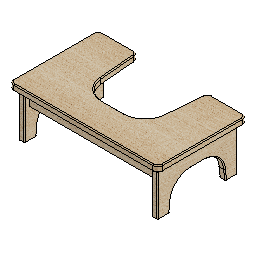
model (Autodesk Fusion 360 design; units mm, degrees)
Autodesk Fusion 360 part; units mm, degrees
sketch "top" plane through (0, 0, 0) normal (0, 0, 1) x (1, 0, 0) in component "stool"
  line L0 (0, 0) -> (500, 0)
  line L1 (150, 100.7611) -> (132.5689, 300)
  line L2 (132.5689, 300) -> (0, 300)
  line L3 (0, 300) -> (0, 0)
  line L4 (150, 100.7611) -> (350, 100.7611)
  line L5 (500, 300) -> (500, 0)
  line L6 (350, 100.7611) -> (367.4311, 300)
  line L7 (367.4311, 300) -> (500, 300)
  arc A0 (285.8568, 100.7611) -> (355.5904, 164.6602) centre (285.8568, 170.7611) ccw
  arc A1 (144.4096, 164.6602) -> (214.1432, 100.7611) centre (214.1432, 170.7611) ccw
  dimension "d5" = 300
  dimension "d6" = 500
  dimension "d7" = 200
  dimension "d8" = 200
  dimension "d21" = 70
  dimension "d36" = 95
  dimension "d37" = 95
  constraint horizontal L0
  constraint horizontal L2
  constraint vertical L3
  constraint coincident L0.start L3.end
  constraint horizontal L4
  constraint vertical L5
  constraint horizontal L7
  constraint equal L2 L7
  constraint equal L3 L5
  constraint tangent L4 A0
  constraint coincident L4 A0.start
  constraint coincident L6 A0.end
  constraint tangent L1 A1
  constraint coincident L1 A1.start
  constraint coincident L4 A1.end
  constraint tangent L6 A0
  constraint tangent L4 A1
  constraint equal A0 A1
  measures "d5" distance of L0.start L2.end
  measures "d6" distance of L0.start L0.end
  measures "d7" distance of L1.start L4.end
  measures "d8" distance of L1.end L1.start
  measures "d21" radius of A0
  measures "d36" angle of L6 L7
  measures "d37" angle of L1 L2
extrude "Extrude1" add sketch "top" along normal blind 21 makes body 1 in component "stool"
sketch "side" plane through (0, 0, 0) normal (1, 0, 0) x (0, 1, 0) in component "stool"
  line L0 (284, 0) -> (284, -150)
  line L1 (284, -150) -> (244, -150)
  line L2 (244, -150) -> (241.0166, -115.8991)
  arc A0 (241.0166, -115.8991) -> (171.2829, -52) centre (171.2829, -122) ccw
  line L3 (171.2829, -52) -> (128.7171, -52)
  arc A1 (128.7171, -52) -> (58.9834, -115.8991) centre (128.7171, -122) ccw
  line L4 (58.9834, -115.8991) -> (56, -150)
  line L5 (56, -150) -> (16, -150)
  line L6 (16, -150) -> (16, 0)
  line L7 (284, 0) -> (16, 0)
  line L8 (150, -52) -> (150, 0) construction
  line L9 (16, 0) -> (0, 0) construction
  point P0 (300, 0)
  dimension "d13" = 16
  dimension "d14" = 16
  dimension "d15" = 40
  dimension "d17" = 150
  dimension "d18" = 70
  dimension "d32" = 52
  dimension "d34" = 95
  dimension "d35" = 95
  constraint tangent L2 A0
  constraint tangent A0 L3
  constraint tangent L3 A1
  constraint tangent A1 L4
  constraint vertical L0
  constraint horizontal L1
  constraint horizontal L3
  constraint horizontal L5
  constraint vertical L6
  constraint equal L1 L5
  constraint equal L0 L6
  constraint equal A0 A1
  constraint perpendicular L6 L7
  constraint midpoint L3 L8.start
  constraint midpoint L7 L8.end
  constraint coincident L9.end origin
  constraint horizontal L9.end L6.end
  measures "d13" distance of P0 L0.start
  measures "d14" distance of L9.end L6.end
  measures "d15" distance of L0.end L1.end
  measures "d17" distance of L0.start L0.end
  measures "d18" radius of A0
  measures "d32" distance of L8.start L8.end
  measures "d34" angle of L1 L2
  measures "d35" angle of L4 L5
extrude "Extrude2" add sketch "side" along normal blind 21 from surface at 16 separate body makes body 2 in component "stool"
ref_plane "WorkPlane1" through (250, 150, 10.5) normal (-1, 0, 0) x (0, -1, 0) in component "stool"
mirror "Mirror1" about plane through (250, 150, 10.5) normal (-1, 0, 0) of bodies 2 makes body 3 in component "stool"
sketch "stretcher" plane through (0, 0, 0) normal (0, 1, 0) x (1, 0, 0) in component "stool"
  line L0 (37, 0) -> (37, 150)
  line L1 (463, 0) -> (463, 150)
  line L2 (37, 0) -> (463, 0)
  line L3 (463, 0) -> (463, 52)
  line L4 (463, 52) -> (37, 52)
  line L5 (37, 52) -> (37, 0)
  dimension "d27" = 52
  constraint horizontal L2
  constraint vertical L3
  constraint horizontal L4
  constraint vertical L5
  constraint coincident L1 L3.end
  constraint coincident L0.start L2.start
  measures "d27" distance of L2 L4
extrude "Extrude3" add sketch "stretcher" along normal blind 21 from surface at 32 separate body makes body 4 in component "stool"
fillet "Fillet1" radius 16 6 edges at (0, 300, 10.5) (0, 0, 10.5) (500, 0, 10.5) (500, 300, 10.5) (132.5689, 300, 10.5) (367.4311, 300, 10.5) on bodies 1 in component "stool"
fillet "Fillet2" radius 3.175 30 edges at (16, 242.5083, -132.9495) (16, 218.5742, -70.3906) (16, 150, -52) (16, 81.4258, -70.3906) (16, 57.4917, -132.9495) (16, 16, -75) (37, 16, -75) (37, 284, -75) (16, 284, -75) (37, 57.4917, -132.9495) (37, 81.4258, -70.3906) (37, 150, -52) (37, 218.5742, -70.3906) (37, 242.5083, -132.9495) (463, 57.4917, -132.9495) (463, 81.4258, -70.3906) (463, 150, -52) (463, 218.5742, -70.3906) (463, 242.5083, -132.9495) (484, 242.5083, -132.9495) (484, 218.5742, -70.3906) (484, 150, -52) (484, 81.4258, -70.3906) (484, 57.4917, -132.9495) (463, 16, -75) (484, 16, -75) (484, 284, -75) (463, 284, -75) (250, 32, -52) (250, 53, -52) 6 faces at (451.8635, 154.8867, 21) (451.8635, 154.8867, 0) (23, 270.6667, -150) (23, 42.6667, -150) (477, 270.6667, -150) (477, 42.6667, -150) on bodies 1 2 3 4 in component "stool"
component "stool" placed x (1, 0, 0) y (0, 1, 0) z (0, 0, 1) at (0, 0, 0)
equation "width = 500 mm"
equation "depth = 300 mm"
equation "holeWidth = 200 mm"
equation "holeDepth = 200 mm"
equation "d5 = depth"
equation "d6 = width"
equation "d7 = holeWidth"
equation "d8 = holeDepth"
equation "thickness = 21 mm"
equation "d10 = thickness"
equation "inset = 16 mm"
equation "d13 = inset"
equation "d14 = d13"
equation "d15 = memberWidth"
equation "height = 150 mm"
equation "d17 = height"
equation "d18 = largeRadius"
equation "memberWidth = 40 mm"
equation "largeRadius = 70 mm"
equation "d21 = largeRadius"
equation "d22 = inset"
equation "d23 = thickness"
equation "d27 = stretcherWidth"
equation "d28 = inset * 2"
equation "d29 = thickness"
equation "stretcherWidth = memberWidth * 1.3"
equation "d32 = stretcherWidth"
equation "taper = 5 deg"
equation "d34 = 90 deg + taper"
equation "d35 = 90 deg + taper"
equation "d36 = 90 deg + taper"
equation "d37 = 90 deg + taper"
equation "d39 = inset"
equation "d41 = 1/8\""
